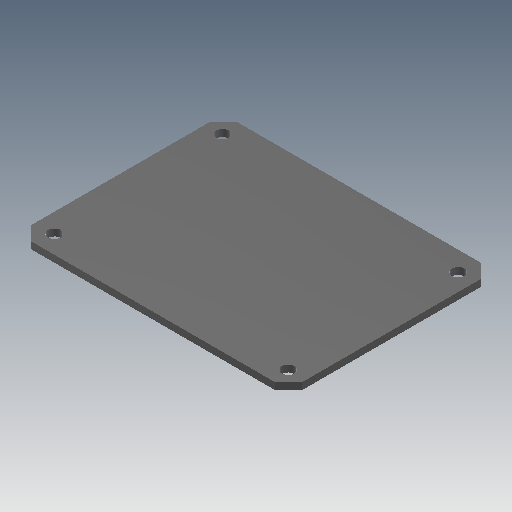
# Autodesk Inventor part: PCB
Saved by Autodesk Inventor 2020 (Build 240168000, 168)
## iProperties
Created: 2019-05-21
Part Number: PCB
Material: ABS Plastic
Document SubType Name: Modeling
Designer: chitl
Density: 1.06 g/cm^3
Appearance: Smooth - White
Mass: 5.11526 g
Surface Area: 64.382 cm^2
Volume: 4.82572 cm^3
Author: chitl
Autodesk Inventor part; units mm, degrees
ref_plane "YZ Plane" through (0, 0, 0) normal (1, 0, 0) x (0, 1, 0)
ref_plane "XZ Plane" through (0, 0, 0) normal (0, 1, 0) x (-1, 0, 0)
ref_plane "XY Plane" through (0, 0, 0) normal (0, 0, 1) x (1, 0, 0)
sketch "Sketch1" plane through (0, 0, 0) normal (0, 1, 0) x (-1, 0, 0)
  line L0 (31.75, 24.13) -> (-31.75, 24.13)
  line L1 (-31.75, 24.13) -> (-31.75, -24.13)
  line L2 (-31.75, -24.13) -> (31.75, -24.13)
  line L3 (31.75, -24.13) -> (31.75, 24.13)
  line L4 (31.75, 24.13) -> (-31.75, -24.13) construction
  line L5 (-31.75, 24.13) -> (31.75, -24.13) construction
  point P0 (0, 0)
  dimension "d0" = 63.5
  dimension "d1" = 48.26
  constraints: 12 end point, 2 midpoint, 2 parallel, 1 horizontal, 1 perpendicular
  measures "d0" distance of L2.end L1.end
  measures "d1" distance of L1.end L0.end
extrude "Extrusion1" add sketch "Sketch1" along normal blind 1.6
chamfer "Chamfer1" distance 3.175 angle 45 4 edges at (31.75, 0.8, 24.13) (31.75, 0.8, -24.13) (-31.75, 0.8, -24.13) (-31.75, 0.8, 24.13)
sketch "Sketch2" plane through (0, 1.6, 0) normal (0, 1, 0) x (1, 0, 0)
  point P0 (0, 0)
  point P1 (-27.7731, 19.9434)
  point P2 (27.7322, 19.5576)
  point P3 (-27.294, -19.8576)
  point P4 (27.5822, -20.0921)
hole "Hole1" at (-27.7731, 1.6, -19.9434) at (27.7322, 1.6, -19.5576) at (-27.294, 1.6, 19.8576) at (27.5822, 1.6, 20.0921) direction (0, -1, 0) diameter 3 depth 95.25 tip angle 118
body "Solid1"
